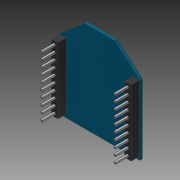
# Autodesk Inventor part: xbee
Saved by Autodesk Inventor 2014 SP2 (Build 180246200, 246)
## iProperties
Created: 2015-03-19
Part Number: xbee
Material: Plastique ABS
Document SubType Name: Modeling
Designer: sd
Density: 1.06 g/cm^3
Appearance: Lisse - Blanc
Mass: 0.528787 g
Surface Area: 13.2375 cm^2
Volume: 0.498855 cm^3
Author: sd
Autodesk Inventor part; units mm, degrees
ref_plane "YZ Plane" through (0, 0, 0) normal (1, 0, 0) x (0, 1, 0)
ref_plane "XZ Plane" through (0, 0, 0) normal (0, 1, 0) x (-1, 0, 0)
ref_plane "XY Plane" through (0, 0, 0) normal (0, 0, 1) x (1, 0, 0)
sketch "Esquisse1" plane through (0, 0, 0) normal (0, 1, 0) x (-1, 0, 0)
  line L0 (-12, -9) -> (12.38, -9)
  line L1 (12.38, -9) -> (12.38, 12.08)
  line L2 (12.38, 12.08) -> (4.79, 18.61)
  line L3 (4.79, 18.61) -> (-4.41, 18.61)
  line L4 (-4.41, 18.61) -> (-12, 12.08)
  line L5 (-12, 12.08) -> (-12, -9)
  point P0 (0, 0)
  dimension "d0" = 24.38
  dimension "d1" = 27.61
  dimension "d2" = 6.53
  dimension "d3" = 6.53
  dimension "d4" = 7.59
  dimension "d5" = 7.59
  dimension "d6" = 24.38
  dimension "d7" = 27.61
  dimension "d8" = 9
  dimension "d9" = 12
  constraints: 12 end point, 1 parallel, 1 perpendicular
  measures "d0" distance of L0.start L0.end
  measures "d1" distance between parallel lines of L0 L3
  measures "d2" vertical distance of L1.end L2.end
  measures "d3" vertical distance of L3.end L4.end
  measures "d4" horizontal distance of L3.end L4.end
  measures "d5" horizontal distance of L1.end L2.end
  measures "d6" distance of L4.end L1.end
  measures "d7" vertical distance of L0.start L3.end
  measures "d8" distance from line of point (0, 0) L0
  measures "d9" distance from line of point (0, 0) L5
extrude "Extrusion1" add sketch "Esquisse1" along normal blind 0.8
sketch "Esquisse2" plane through (0, 0, 0) normal (0, -1, 0) x (1, 0, 0)
  line L0 (12, -9) -> (-12.38, -9) projected
  line L1 (-12.28, 12) -> (-10.28, 12)
  line L2 (-10.28, 12) -> (-10.28, -8)
  line L3 (-10.28, -8) -> (-12.28, -8)
  line L4 (-12.28, -8) -> (-12.28, 12)
  line L5 (9.9, 12) -> (11.9, 12)
  line L6 (11.9, 12) -> (11.9, -8)
  line L7 (11.9, -8) -> (9.9, -8)
  line L8 (9.9, -8) -> (9.9, 12)
  point P0 (12, 12.08)
  point P1 (-12.38, 12.08)
  point P2 (0, 0)
  dimension "d12" = 2
  dimension "d13" = 2
  dimension "d14" = 20
  dimension "d15" = 20
  dimension "d16" = 1
  dimension "d17" = 1
  dimension "d18" = 0.1
  dimension "d19" = 0.1
  constraints: 16 end point, 4 parallel, 2 horizontal, 2 perpendicular
  measures "d12" distance of L1.start L1.end
  measures "d13" distance of L5.start L5.end
  measures "d14" distance of L5.end L6.end
  measures "d15" distance of L3.end L1.start
  measures "d16" distance between parallel lines of L0 L3
  measures "d17" distance between parallel lines of L0 L7
  measures "d18" distance from line of point (-12.38, 12.08) L4
  measures "d19" horizontal distance of point (12, 12.08) L5.end
extrude "Extrusion2" add sketch "Esquisse2" along normal blind 2.5
sketch "Esquisse3" plane through (0, -2.5, 0) normal (0, -1, 0) x (1, 0, 0)
  line L0 (-10.28, 12) -> (-12.28, 12) projected
  line L1 (-12.28, 12) -> (-12.28, -8) projected
  line L2 (-11.535, 11.255) -> (-11.025, 11.255)
  line L3 (-11.025, 11.255) -> (-11.025, 10.745)
  line L4 (-11.025, 10.745) -> (-11.535, 10.745)
  line L5 (-11.535, 10.745) -> (-11.535, 11.255)
  line L6 (10.645, 11.255) -> (11.155, 11.255)
  line L7 (11.155, 11.255) -> (11.155, 10.745)
  line L8 (11.155, 10.745) -> (10.645, 10.745)
  line L9 (10.645, 10.745) -> (10.645, 11.255)
  line L10 (11.9, 12) -> (9.9, 12) projected
  line L11 (9.9, 12) -> (9.9, -8) projected
  point P0 (0, 0)
  dimension "d22" = 0.51
  dimension "d23" = 0.51
  dimension "d24" = 20
  dimension "d25" = 0.745
  dimension "d26" = 0.745
  dimension "d27" = 2
  dimension "d28" = 0.51
  dimension "d29" = 0.51
  dimension "d30" = 0.745
  dimension "d31" = 0.745
  constraints: 16 end point, 4 parallel, 2 horizontal, 2 perpendicular
  measures "d22" distance of L2.start L2.end
  measures "d23" distance of L4.end L2.start
  measures "d24" distance of L0.end L1.end
  measures "d25" distance between parallel lines of L0 L2
  measures "d26" distance between parallel lines of L1 L5
  measures "d27" distance of L0.start L0.end
  measures "d28" distance of L6.start L6.end
  measures "d29" distance of L8.end L6.start
  measures "d30" distance between parallel lines of L10 L6
  measures "d31" distance between parallel lines of L11 L9
extrude "Extrusion3" add sketch "Esquisse3" along normal blind 4.06
chamfer "Chanfrein1" distance 0.1 angle 45 8 edges at (-11.28, -6.56, 11.255) (-11.535, -6.56, 11) (-11.28, -6.56, 10.745) (-11.025, -6.56, 11) (10.9, -6.56, 11.255) (10.645, -6.56, 11) (10.9, -6.56, 10.745) (11.155, -6.56, 11)
pattern_linear "Réseau rectangulaire1" count 10 spacing 2 along (0, 0, -1) of "Extrusion3", "Chanfrein1"
equation "\"d3\" = d2"
equation "\"d5\" = d4"
equation "\"d6\" = d0"
equation "\"d7\" = d1"
equation "\"d13\" = d12"
equation "\"d15\" = d14"
equation "\"d17\" = d16"
equation "\"d19\" = d18"
equation "\"d23\" = d22"
equation "\"d26\" = -0.5 * d22 + 0.5 * d27"
equation "\"d28\" = d22"
equation "\"d29\" = d23"
equation "\"d30\" = d25"
equation "\"d31\" = d26"
